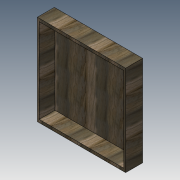
# Autodesk Inventor part: FLY MEDIA CARDBOARD TRAY
Saved by Autodesk Inventor 2018.3 (Build 223284000, 284)
## iProperties
Created: 2018-09-09
Material: Generic
Vendor: HHMI: JRC - ID&F
Document SubType Name: Modeling
Designer: arnoldj
Density: 1 g/cm^3
Appearance: Driftwood
RuleStatus: InUse
AfterDocSave0: file://Part Number Cleaner
DESIGN DEPARTMENT: HHMI: JRC - ID&F
ALTERED ITEM PART NUMBER: N/A
ALTERED ITEM VENDOR: N/A
ALTERED ITEM DESCRIPTION: N/A
Author: arnoldj
Revision Number: 0
Autodesk Inventor part; units mm, degrees
ref_plane "YZ Plane" through (0, 0, 0) normal (1, 0, 0) x (0, 1, 0)
ref_plane "XZ Plane" through (0, 0, 0) normal (0, 1, 0) x (-1, 0, 0)
ref_plane "XY Plane" through (0, 0, 0) normal (0, 0, 1) x (1, 0, 0)
sketch "Sketch1" plane through (0, 0, 0) normal (0, 0, 1) x (1, 0, 0)
  line L0 (0, 215.5825) -> (0, -215.5825) projected
  line L1 (-210.49, 0) -> (210.49, 0) projected
  line L2 (144, -144) -> (-144, -144)
  line L3 (-144, -144) -> (-144, 144)
  line L4 (-144, 144) -> (144, 144)
  line L5 (144, 144) -> (144, -144)
  line L6 (144, -144) -> (-144, 144) construction
  line L7 (-144, -144) -> (144, 144) construction
  line L8 (150.35, 153.9875) -> (-150.35, 153.9875)
  line L9 (-150.35, 153.9875) -> (-150.35, -153.9875)
  line L10 (-150.35, -153.9875) -> (150.35, -153.9875)
  line L11 (150.35, -153.9875) -> (150.35, 153.9875)
  point P0 (0, 0)
  dimension "d0" = 288
  dimension "d6" = 6.35
  dimension "d7" = 6.35
  dimension "d8" = 9.9875
  dimension "d9" = 307.975
  dimension "d10" = 9.9875
  constraints: 20 end point, 4 parallel, 3 perpendicular, 2 midpoint, 1 horizontal
  measures "d0" distance of L3.end L4.end
  measures "d6" distance between parallel lines of L9 L3
  measures "d7" distance between parallel lines of L11 L5
  measures "d8" distance between parallel lines of L8 L4
  measures "d9" distance of L8.end L9.end
  measures "d10" distance between parallel lines of L2 L10
extrude "Extrusion1" add sketch "Sketch1" along normal blind 53.594 contours L8 L11 L1 L5 L4 L0 | L0 L4 L3 L1 L9 L8 | L11 L10 L0 L2 L5 L1 | L1 L3 L2 L0 L10 L9
sketch "Sketch2" plane through (0, 0, 0) normal (0, 0, -1) x (-1, 0, 0)
  line L0 (144, 144) -> (144, -144) projected
  line L1 (144, -144) -> (-144, -144) projected
  line L2 (-144, -144) -> (-144, 144) projected
  line L3 (-144, 144) -> (144, 144) projected
  line L4 (-150.35, 153.9875) -> (150.35, 153.9875) projected
  line L5 (-150.35, -153.9875) -> (-150.35, 153.9875) projected
  line L6 (150.35, -153.9875) -> (-150.35, -153.9875) projected
  line L7 (150.35, 153.9875) -> (150.35, -153.9875) projected
  point P0 (0, 0)
extrude "Extrusion2" add sketch "Sketch2" along normal blind 4.445 contours L0 L1 L2 L3 | L4 L7 L6 L5
equation "\"d8\" = d10"
body "Solid1"
